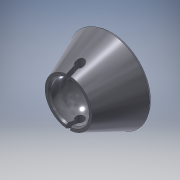
# Autodesk Inventor part: Table Clamp Swiveling Pad
Saved by Autodesk Inventor 2016 (Build 200138000, 138)
## iProperties
Created: 2017-11-17
Part Number: Table Clamp Swiveling Pad
Material: SAE 1020
Document SubType Name: Modeling
Designer: Zigunov
Stock Number: 0
Mass: 1729.01 g
Surface Area: 745.421 cm^2
Volume: 219.697 cm^3
Density: 7.87 g/cm^3
Appearance: Steel - Polished
Author: Zigunov
Autodesk Inventor part; units mm, degrees
ref_plane "YZ Plane" through (0, 0, 0) normal (1, 0, 0) x (0, 1, 0)
ref_plane "XZ Plane" through (0, 0, 0) normal (0, 1, 0) x (-1, 0, 0)
ref_plane "XY Plane" through (0, 0, 0) normal (0, 0, 1) x (1, 0, 0)
sketch "Sketch2" plane through (0, 0, 0) normal (0, 0, 1) x (1, 0, 0)
  arc A0 (3.5799, -1.6693) -> (1.25, 3.747) centre (0, 0) ccw
  line L0 (3.5799, -1.6693) -> (4.51, -1.6693)
  line L1 (4.51, -1.6693) -> (7.8046, 6.0923)
  line L2 (7.5, 6.5525) -> (0, 6.5525)
  line L3 (0, 6.5525) -> (0, 4.5525)
  arc A1 (0, 4.5525) -> (1.25, 3.747) centre (2.1994, 6.5928) ccw
  line L4 (0, 0) -> (1.25, 0) construction
  line L5 (7.8046, 6.0923) -> (7.5, 6.5525)
  point P0 (8, 6.5525)
  dimension "d11" = 3.95
  dimension "d12" = 2
  dimension "d13" = 67
  dimension "d14" = 3
  dimension "d15" = 2.5
  dimension "d16" = 25
  dimension "d17" = 0.5
  dimension "d18" = 0.5
  dimension "d19" = 16
  dimension "d20" = 0.9301
  constraints: 12 end point, 4 point on circle, 3 point on line, 2 centre point, 2 horizontal, 1 coincident, 1 parallel, 1 tangent, 1 vertical
  measures "d11" radius of A0
  measures "d12" distance of L2.end L3.end
  measures "d13" angle of L1 L2
  measures "d14" radius of A1
  measures "d15" diameter of A0.end L3
  measures "d17" distance of L1.end point (8, 6.553)
  measures "d18" distance of L2.start point (8, 6.553)
  measures "d19" diameter of point (8, 6.553) L3
  measures "d20" distance of L0.start L0.end
revolve "Revolution1" add sketch "Sketch2" angle 360 about axis through (0, 6.5525, 0) along (0, -1, 0)
chamfer "Chamfer1" distance 0.4 angle 45 1 edges at (-3.5799, -1.6693, 0)
sketch "Sketch3" plane through (0, 0, 0) normal (0, 0, 1) x (1, 0, 0)
  arc A0 (3.7304, -1.2987) -> (-3.7304, -1.2987) centre (0, 0) ccw projected
  line L0 (-3.9799, -1.6693) -> (3.9799, -1.6693) projected
  line L1 (-0.4, -1.6693) -> (0.4, -1.6693)
  line L2 (0.4, -1.6693) -> (0.4, -0.1928)
  line L3 (0.4, -0.1928) -> (-0.4, -0.1928) construction
  line L4 (-0.4, -0.1928) -> (-0.4, -1.6693)
  line L5 (-0.4, -1.6693) -> (0.4, -0.1928) construction
  line L6 (0.4, -1.6693) -> (-0.4, -0.1928) construction
  arc A1 (0.4, -0.1928) -> (-0.4, -0.1928) centre (0, 0.5) ccw
  point P0 (0, -0.9311)
  dimension "d25" = 0.8
  dimension "d26" = 0.8
  dimension "d27" = 0.5
  constraints: 12 end point, 2 midpoint, 2 parallel, 2 point on circle, 1 centre point, 1 horizontal, 1 perpendicular, 1 point on line, 1 vertical alignment
  measures "d25" distance between parallel lines of L4 L2
  measures "d26" radius of A1
  measures "d27" distance of point (0, 0) A1.centre
extrude "Extrusion2" cut sketch "Sketch3" along normal through all both and the other way through all
equation "\"d18\" = d17"
body "Solid2"
